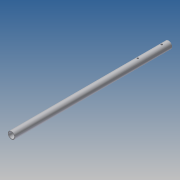
# Autodesk Inventor part: feed-bppvcarm
Saved by Autodesk Inventor 2013 SP2 (Build 170200200, 200)
## iProperties
Company: HERA Project
Created: 2013-07-11
Part Number: feed-bppvcarm
Material: PVC-Piping
Description: PVC arm for feed backplane
Document SubType Name: Modeling
Designer: David DeBoer
Mass: 584.983 g
Surface Area: 2150.15 cm^2
Volume: 417.845 cm^3
Density: 1.4 g/cm^3
Title: feed-bppvcarm
Author: David DeBoer
Autodesk Inventor part; units mm, degrees
ref_plane "YZ Plane" through (0, 0, 0) normal (1, 0, 0) x (0, 1, 0)
ref_plane "XZ Plane" through (0, 0, 0) normal (0, 1, 0) x (-1, 0, 0)
ref_plane "XY Plane" through (0, 0, 0) normal (0, 0, 1) x (1, 0, 0)
sketch "Sketch1" plane through (0, 0, 0) normal (0, 0, 1) x (1, 0, 0)
  circle A0 centre (0, 0) radius 13.335
  circle A1 centre (0, 0) radius 10.4648
  dimension "d0" = 26.67
  dimension "d2" = 2.8702
  constraints: 2 centre point, 1 coincident
  measures "d0" diameter of A0
  measures "d2" radial gap between concentric circles of A1 A0
extrude "Extrusion1" add sketch "Sketch1" along normal blind 584.2
sketch "Sketch2" plane through (0, 0, 584.2) normal (0, 0, 1) x (1, 0, 0)
  circle A0 centre (0, 0) radius 10.4648 projected
  circle A1 centre (0, 0) radius 13.335 projected
  point P0 (0, 13.335)
  constraints: 1 vertical alignment, 1 other
ref_plane "Work Plane1" through (0, 13.335, 584.2) normal (0, 1, 0) x (-1, 0, 0)
sketch "Sketch3" plane through (0, 13.335, 584.2) normal (0, 1, 0) x (-1, 0, 0)
  circle A0 centre (0, -558.8) radius 7.0778
  circle A1 centre (0, -469.9) radius 7.2132
  point P0 (0, -584.2)
  dimension "d5" = 25.4
  dimension "d6" = 88.9
  constraints: 2 centre point
  measures "d5" distance of A0.centre point (0, -584.2)
  measures "d6" distance of A1.centre A0.centre
hole "Hole1" at (0, 13.335, 114.3) at (0, 13.335, 25.4) direction (0, -1, 0) diameter 6.7564 end through all clearance for "Flat Head Machine Screw (82)" size "1/4" standard "Ansi Unified Screw Threads"
body "Solid1"
